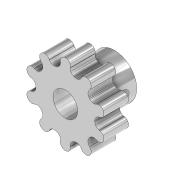
# Autodesk Inventor part: 4th Axis Main Drive Gear
Saved by Autodesk Inventor 2020 (Build 240168000, 168)
## iProperties
Created: 2021-06-28
Part Number: 4th Axis Main Drive Gear
Material: Generic
Document SubType Name: Modeling
Designer: Coy
Density: 1 g/cm^3
Appearance: Chrome - Polished
Author: Coy
Autodesk Inventor part; units mm, degrees
ref_plane "YZ Plane" through (0, 0, 0) normal (1, 0, 0) x (0, 1, 0)
ref_plane "XZ Plane" through (0, 0, 0) normal (0, 1, 0) x (-1, 0, 0)
ref_plane "XY Plane" through (0, 0, 0) normal (0, 0, 1) x (1, 0, 0)
sketch "Sketch4" plane through (0, 0, 0) normal (0, 0, 1) x (1, 0, 0)
  circle A0 centre (0, 0) radius 2.5
  circle A1 centre (0, 0) radius 8.2 construction
  circle A2 centre (0, 0) radius 6
  arc A3 (1.0386, 6.9958) -> (-1.0386, 6.9958) centre (0, 7.15) ccw
  arc A4 (-1.7552, 5.7375) -> (-1.0238, 6.8958) centre (-2.0624, 6.7416) ccw
  arc A5 (1.0238, 6.8958) -> (1.7552, 5.7375) centre (2.0624, 6.7416) ccw
  line L0 (1.0238, 6.8958) -> (1.0386, 6.9958)
  line L1 (-1.0238, 6.8958) -> (-1.0386, 6.9958)
  line L2 (0, 0) -> (0, 6.1) construction
  line L3 (0, 8.2) -> (0, 9.5985) construction
  arc A6 (-3.2718, 6.2702) -> (-4.9523, 5.0492) centre (-4.2027, 5.7845) ccw
  line L4 (-4.8815, 4.9771) -> (-4.9523, 5.0492)
  arc A7 (-4.7924, 3.6101) -> (-4.8815, 4.9771) centre (-5.6311, 4.2418) ccw
  line L5 (-3.225, 6.1806) -> (-3.2718, 6.2702)
  arc A8 (-3.225, 6.1806) -> (-1.9524, 5.6734) centre (-2.2941, 6.6663) ccw
  arc A9 (-6.3325, 3.1496) -> (-6.9744, 1.174) centre (-6.8001, 2.2095) ccw
  line L6 (-6.8746, 1.1573) -> (-6.9744, 1.174)
  arc A10 (-5.9991, 0.1037) -> (-6.8746, 1.1573) centre (-7.0489, 0.1218) ccw
  line L7 (-6.2419, 3.1046) -> (-6.3325, 3.1496)
  arc A11 (-6.2419, 3.1046) -> (-4.9143, 3.4423) centre (-5.7743, 4.0447) ccw
  arc A12 (-6.9744, -1.174) -> (-6.3325, -3.1496) centre (-6.8001, -2.2095) ccw
  line L8 (-6.2419, -3.1046) -> (-6.3325, -3.1496)
  arc A13 (-4.9143, -3.4423) -> (-6.2419, -3.1046) centre (-5.7743, -4.0447) ccw
  line L9 (-6.8746, -1.1573) -> (-6.9744, -1.174)
  arc A14 (-6.8746, -1.1573) -> (-5.9991, -0.1037) centre (-7.0489, -0.1218) ccw
  arc A15 (-4.9523, -5.0492) -> (-3.2718, -6.2702) centre (-4.2027, -5.7845) ccw
  line L10 (-3.225, -6.1806) -> (-3.2718, -6.2702)
  arc A16 (-1.9524, -5.6734) -> (-3.225, -6.1806) centre (-2.2941, -6.6663) ccw
  line L11 (-4.8815, -4.9771) -> (-4.9523, -5.0492)
  arc A17 (-4.8815, -4.9771) -> (-4.7924, -3.6101) centre (-5.6311, -4.2418) ccw
  arc A18 (-1.0386, -6.9958) -> (1.0386, -6.9958) centre (0, -7.15) ccw
  line L12 (1.0238, -6.8958) -> (1.0386, -6.9958)
  arc A19 (1.7552, -5.7375) -> (1.0238, -6.8958) centre (2.0624, -6.7416) ccw
  line L13 (-1.0238, -6.8958) -> (-1.0386, -6.9958)
  arc A20 (-1.0238, -6.8958) -> (-1.7552, -5.7375) centre (-2.0624, -6.7416) ccw
  arc A21 (3.2718, -6.2702) -> (4.9523, -5.0492) centre (4.2027, -5.7845) ccw
  line L14 (4.8815, -4.9771) -> (4.9523, -5.0492)
  arc A22 (4.7924, -3.6101) -> (4.8815, -4.9771) centre (5.6311, -4.2418) ccw
  line L15 (3.225, -6.1806) -> (3.2718, -6.2702)
  arc A23 (3.225, -6.1806) -> (1.9524, -5.6734) centre (2.2941, -6.6663) ccw
  arc A24 (6.3325, -3.1496) -> (6.9744, -1.174) centre (6.8001, -2.2095) ccw
  line L16 (6.8746, -1.1573) -> (6.9744, -1.174)
  arc A25 (5.9991, -0.1037) -> (6.8746, -1.1573) centre (7.0489, -0.1218) ccw
  line L17 (6.2419, -3.1046) -> (6.3325, -3.1496)
  arc A26 (6.2419, -3.1046) -> (4.9143, -3.4423) centre (5.7743, -4.0447) ccw
  arc A27 (6.9744, 1.174) -> (6.3325, 3.1496) centre (6.8001, 2.2095) ccw
  line L18 (6.2419, 3.1046) -> (6.3325, 3.1496)
  arc A28 (4.9143, 3.4423) -> (6.2419, 3.1046) centre (5.7743, 4.0447) ccw
  line L19 (6.8746, 1.1573) -> (6.9744, 1.174)
  arc A29 (6.8746, 1.1573) -> (5.9991, 0.1037) centre (7.0489, 0.1218) ccw
  arc A30 (4.9523, 5.0492) -> (3.2718, 6.2702) centre (4.2027, 5.7845) ccw
  line L20 (3.225, 6.1806) -> (3.2718, 6.2702)
  arc A31 (1.9524, 5.6734) -> (3.225, 6.1806) centre (2.2941, 6.6663) ccw
  line L21 (4.8815, 4.9771) -> (4.9523, 5.0492)
  arc A32 (4.8815, 4.9771) -> (4.7924, 3.6101) centre (5.6311, 4.2418) ccw
  point P0 (-4.8198, 6.6339)
  point P1 (-7.7987, 2.5339)
  point P2 (-7.7987, -2.5339)
  point P3 (-4.8198, -6.6339)
  point P4 (0, -8.2)
  point P5 (4.8198, -6.6339)
  point P6 (7.7987, -2.5339)
  point P7 (7.7987, 2.5339)
  point P8 (4.8198, 6.6339)
  point P9 (-4.9143, 3.4423)
  point P10 (-5.9991, -0.1037)
  point P11 (-1.9524, -5.6734)
  point P12 (1.9524, -5.6734)
  point P13 (4.9143, -3.4423)
  point P14 (5.9991, 0.1037)
  dimension "d19" = 5
  dimension "d20" = 16.4
  dimension "d21" = 2.2
  dimension "d22" = 2.1
  dimension "d23" = 2.1
  dimension "d24" = 2.1
  dimension "d27" = 360
  constraints: 72 point on circle, 44 end point, 33 centre point, 7 tangent, 2 coincident, 2 line through centre, 2 vertical, 151 other
  measures "d19" diameter of A0
  measures "d20" diameter of A1
  measures "d21" radial gap between concentric circles of A1 A2
  measures "d22" diameter of A3
  measures "d23" diameter of A5
  measures "d24" diameter of A4
extrude "Extrusion4" add sketch "Sketch4" along normal blind 5
sketch "Sketch5" plane through (0, 0, 0) normal (0, 0, -1) x (-1, 0, 0)
  circle A0 centre (0, 0) radius 2.5
  circle A1 centre (0, 0) radius 4.5
  dimension "d31" = 2
  constraints: 2 centre point, 1 coincident
  measures "d31" radial gap between concentric circles of A0 A1
extrude "Extrusion5" add sketch "Sketch5" along normal blind 5
sketch "Sketch6" plane through (0, 0, 0) normal (1, 0, 0) x (0, 1, 0)
  line L0 (4.5, 0) -> (4.5, -5) projected
  line L1 (4.5, -2.5) -> (-4.5, -2.5) construction
  line L2 (-4.5, 0) -> (-4.5, -5) construction
  circle A0 centre (0, -2.5) radius 0.95
  point P0 (0, 0)
  dimension "d34" = 1.9
  constraints: 3 midpoint, 2 end point, 1 centre point
  measures "d34" diameter of A0
extrude "Extrusion6" cut sketch "Sketch6" against normal through all both and the other way through all
equation "\"d23\" = d22"
equation "\"d24\" = d22"
body "Solid2"
